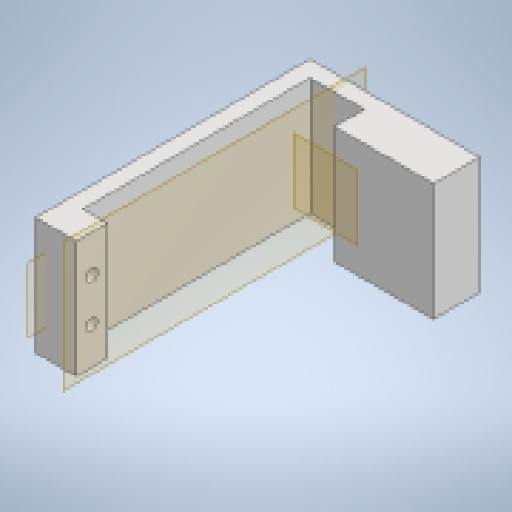
# Autodesk Inventor part: Base Side Armor - Right
Saved by Autodesk Inventor 2023 (Build 270158000, 158)
## iProperties
Created: 2024-09-28
Part Number: Base Side Armor - Right
Material: Generic
Document SubType Name: Modeling
Designer: Ethan
Density: 1 g/cm^3
Appearance: Default
Author: Ethan
Autodesk Inventor part; units mm, degrees
ref_plane "XZ Plane" through (0, 0, 0) normal (0, 1, 0) x (-1, 0, 0)
ref_plane "Back of Base Plane" through (0, 0, -65.3556) normal (0, 0, 1) x (1, 0, 0)
ref_plane "Side of Base Plane" through (-6.5, 0, 0) normal (1, 0, 0) x (0, 1, 0)
ref_plane "Side Bolt Offset Plane" through (-16.2, 0, 0) normal (1, 0, 0) x (0, 1, 0)
ref_plane "Back Bolt Offset Plane" through (0, 0, -75.3556) normal (0, 0, 1) x (1, 0, 0)
sketch "Interface-EDIT TO CHANGE SHAPE" plane through (0, 0, 0) normal (0, 1, 0) x (-1, 0, 0)
  line L0 (0, 0) -> (14, 0) construction
  line L1 (14, 0) -> (14, -74.5296) construction
  line L2 (14, -74.5296) -> (-27.5, -74.5296) construction
  line L3 (-27.5, -74.5296) -> (-27.5, -65.3556) construction
  line L4 (-46.4, -65.3556) -> (29.9, -65.3556) construction
  line L5 (14, -4.75) -> (14, -74.5296)
  line L6 (14, -74.5296) -> (-2.7, -74.5296)
  line L7 (-2.7, -74.5296) -> (-2.7, -65.3556)
  line L8 (19, 4.75) -> (19, -79.5296)
  line L9 (19, -79.5296) -> (-35.5, -79.5296)
  line L10 (-35.5, -79.5296) -> (-35.5, -65.3556)
  line L11 (0, -96.3855) -> (0, 21.6059) construction
  line L12 (14, -4.75) -> (6.5, -4.75)
  line L13 (19, 4.75) -> (6.5, 4.75)
  line L14 (6.5, 4.75) -> (6.5, -4.75)
  line L15 (6.5, -96.3855) -> (6.5, 21.6059) construction
  line L16 (-2.7, -65.3556) -> (-35.5, -65.3556)
  dimension "d8" = -27.5
  dimension "d9" = 9.5
  dimension "d10" = 9.174
  dimension "d11" = -14
  dimension "d14" = -5
  dimension "d15" = 5
  dimension "d33" = -24.8
  dimension "d34" = -8
  constraints: 28 end point, 7 perpendicular, 4 collinear, 4 horizontal, 1 point on line, 1 vertical, 1 other
  measures "d8" distance between parallel lines of L11 L3
  measures "d9" distance of L13.end L12.end
  measures "d10" distance between parallel lines of L4 L2
  measures "d11" distance between parallel lines of L1 L11
  measures "d14" distance between parallel lines of L8 L5
  measures "d15" distance between parallel lines of L9 L6
  measures "d33" distance between parallel lines of L7 L3
  measures "d34" distance between parallel lines of L3 L10
extrude "Interface-EDIT TO CHANGE MOUNT HEIGHT" add sketch "Interface-EDIT TO CHANGE SHAPE" along normal mid plane 40
sketch "Side Bolt Shaft Holes Sketch" plane through (-16.2, 0, 0) normal (1, 0, 0) x (0, 1, 0)
  circle A0 centre (6.5, 0) radius 1.75
  circle A1 centre (-6.5, 0) radius 1.75
  line L0 (6.5, 0) -> (-6.5, 0) construction
  point P0 (0, 0)
  point P1 (0, 0)
  dimension "d18" = 6.5
  dimension "d19" = 3.5
  constraints: 3 coincident, 2 centre point, 2 end point, 1 equal radius, 1 horizontal, 1 midpoint
  measures "d18" distance of point (0, 0) A0.centre
  measures "d19" diameter of A0
extrude "Bolt Shaft Holes - Side" cut sketch "Side Bolt Shaft Holes Sketch" along normal through all both and the other way through all
sketch "Side Bolt Head Holes Sketch" plane through (-16.2, 0, 0) normal (1, 0, 0) x (0, 1, 0)
  circle A0 centre (6.5, 0) radius 1.75 projected
  circle A1 centre (6.5, 0) radius 3.25
  circle A2 centre (-6.5, 0) radius 1.75 projected
  circle A3 centre (-6.5, 0) radius 3.25
  point P0 (0, 0)
  dimension "d22" = 6.5
  constraints: 2 centre point, 2 coincident, 1 equal radius
  measures "d22" diameter of A1
extrude "Bolt Head Holes - Side" cut sketch "Side Bolt Head Holes Sketch" against normal through all contours A0 | A1 | A2 | A3
sketch "Back Bolt Shaft Holes Sketch" plane through (0, 0, -75.3556) normal (0, 0, 1) x (1, 0, 0)
  line L0 (27.5, 6.5) -> (27.5, -6.5) construction
  circle A0 centre (27.5, 6.5) radius 1.75
  circle A1 centre (27.5, -6.5) radius 1.75
  point P0 (0, 0)
  point P1 (27.5, 0)
  point P2 (27.5, 0)
  point P3 (27.5, 0)
  point P4 (27.5, 0)
  dimension "d25" = 6.5
  dimension "d26" = 3.5
  constraints: 3 coincident, 2 centre point, 2 end point, 1 equal radius, 1 midpoint, 1 vertical
  measures "d25" distance of point (27.5, 0) L0.start
  measures "d26" diameter of A0
extrude "Back Bolt Shaft Holes" cut sketch "Back Bolt Shaft Holes Sketch" along normal through all both and the other way through all
sketch "Back Bolt Head Holes Sketch" plane through (0, 0, -75.3556) normal (0, 0, 1) x (1, 0, 0)
  circle A0 centre (27.5, 6.5) radius 1.75 projected
  circle A1 centre (27.5, 6.5) radius 3.25
  circle A2 centre (27.5, -6.5) radius 3.25
  point P0 (0, 0)
  dimension "d29" = 6.5
  constraints: 2 centre point, 2 coincident, 1 equal radius
  measures "d29" diameter of A1
extrude "Back Bolt Head Holes" cut sketch "Back Bolt Head Holes Sketch" against normal through all contours A0 | A1 | A2
fillet "Mount Fillets" radius 2 4 edges at (-10.25, 20, -4.75) (-10.25, -20, -4.75) (2.7, -20, -69.9426) (2.7, 20, -69.9426)
fillet "Internal Fillets" radius 3 7 edges at (-14, 19.4142, -4.1642) (-14, -19.4142, -4.1642) (-14, 0, -4.75) (-14, 0, -74.5296) (3.2858, 19.4142, -74.5296) (3.2858, -19.4142, -74.5296) (2.7, 0, -74.5296)
body "Solid2"
